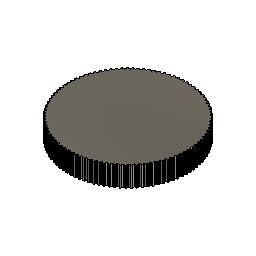
gear_95z (Autodesk Fusion 360 design; units mm, degrees)
Autodesk Fusion 360 part; units mm, degrees
sketch "Sketch1" plane through (0, 0, 0) normal (0, 0, 1) x (1, 0, 0) in component "gt2 pulley"
  circle A0 centre (0, 0) radius 30.2394 construction
  circle A1 centre (0, 0) radius 29.2354 construction
  line L0 (0, 0) -> (0, 30.2394) construction
  line L1 (0, 0) -> (0.9998, 30.2229) construction
  line L2 (0, 0) -> (1.4042, 30.2068) construction
  circle A2 centre (0, 0) radius 29.9854 construction
  arc A3 (0.3977, 29.8499) -> (0.4768, 29.551) centre (1.3924, 29.9531) ccw
  circle A4 centre (0, 0) radius 29.8354 construction
  arc A5 (0.2497, 29.9844) -> (0, 29.9854) centre (0, 0) ccw
  arc A6 (0.3977, 29.8499) -> (0.2497, 29.9844) centre (0.2486, 29.8344) ccw
  arc A7 (0.4768, 29.551) -> (0.9666, 29.2195) centre (0.985, 29.7742) ccw
  arc A8 (0, 29.9854) -> (-0.2497, 29.9844) centre (0, 0) ccw
  arc A9 (-0.2497, 29.9844) -> (-0.3977, 29.8499) centre (-0.2486, 29.8344) ccw
  arc A10 (-0.4768, 29.551) -> (-0.3977, 29.8499) centre (-1.3924, 29.9531) ccw
  arc A11 (-0.9669, 29.2194) -> (-0.4768, 29.551) centre (-0.985, 29.7742) ccw
  arc A12 (0.9666, 29.2195) -> (-0.9666, 29.2195) centre (0, 0) ccw
  point P0 (1.3924, 29.9531)
  point P1 (0, 29.9854)
  dimension "d18" = 60.4789
  dimension "d19" = 1.895
  dimension "d22" = 1.004
  dimension "d24" = 0.75
  dimension "d26" = 1
  dimension "d27" = 0.15
  dimension "d28" = 0.15
  dimension "d47" = 0.555
  dimension "d52" = 3.812
  constraint coincident A0.centre A1.centre
  constraint coincident A0 L0.end
  constraint vertical L0
  constraint coincident A0 L1.end
  constraint coincident A0 L2.end
  constraint concentric A1 A2
  constraint coincident A1 A7.end
  constraint coincident L1 A7.end
  constraint coincident A2 P0
  constraint coincident L2 P0
  constraint coincident P0 A3.centre
  constraint coincident A2 P1
  constraint coincident L0 P1
  constraint concentric A2 A4
  constraint coincident P1 A5.end
  constraint coincident A4 A6.centre
  constraint coincident A3.start A6.start
  constraint tangent A3 A6
  constraint tangent A3 A7
  constraint symmetric L0 A7.end A12.end
  constraint symmetric L0 A3.start A9.end
  constraint symmetric L0 A3.end A10.start
  constraint symmetric L0 A3 A10
  constraint symmetric L0 A5.start A8.end
  constraint symmetric L0 P1 A5.end
  constraint symmetric L0 A5 A8
  constraint symmetric L0 A6 A9
  constraint symmetric L0 A7 A11
  constraint coincident A1 A11.start
  constraint tangent A1 A7
  constraint coincident L1 A7.centre
  measures "d18" diameter of A0
  measures "d19" angle of L0 L1
  measures "d22" distance of A0 A1
  measures "d24" distance of A1 A2
  measures "d26" radius of A3
  measures "d27" distance of A2 A4
  measures "d28" radius of A6
  measures "d47" radius of A7
extrude "Extrude1" add sketch "Sketch1" along normal blind 10 makes body 1
pattern_circular "C-Pattern1" count 95 over 360 about axis through (0, 0, 1.75) along (0, 0, 1) of bodies 1 makes body 2 at (-2.0395, 29.1642, 6.6667) makes body 3 at (-3.1094, 29.0696, 6.6667) makes body 4 at (-6.4983, 28.5041, 6.6667) makes body 5 at (-7.5409, 28.2462, 6.6667) makes body 6 at (-8.7785, 27.8864, 3.3333) makes body 7 at (-11.9894, 26.6639, 6.6667) makes body 8 at (-12.3798, 26.4849, 3.3333) makes body 9 at (-14.6643, 25.2917, 6.6667) makes body 10 at (-16.4817, 24.1467, 6.6667) makes body 11 at (-18.5444, 22.6013, 6.6667) makes body 12 at (-19.9976, 21.3262, 6.6667) makes body 13 at (-20.3087, 21.0302, 3.3333) makes body 14 at (-22.2222, 18.997, 6.6667) makes body 15 at (-22.905, 18.1679, 6.6667) makes body 16 at (-24.0556, 16.6144, 3.3333) makes body 17 at (-25.8387, 13.6775, 6.6667) makes body 18 at (-26.4164, 12.5254, 6.6667) makes body 19 at (-27.4169, 10.1501, 6.6667) makes body 20 at (-27.9659, 8.5217, 6.6667) makes body 21 at (-28.1469, 7.9033, 3.3333) makes body 22 at (-28.6077, 6.0258, 3.3333) makes body 23 at (-29.1171, 2.628, 6.6667) makes body 24 at (-29.2271, 0.6979, 6.6667) makes body 25 at (-29.2342, 0.2685, 6.6667) makes body 26 at (-29.1265, -2.5214, 6.6667) makes body 27 at (-29.0142, -3.5896, 3.3333) makes body 28 at (-28.7136, -5.4993, 3.3333) makes body 29 at (-27.8701, -8.8299, 6.6667) makes body 30 at (-27.7374, -9.2384, 3.3333) makes body 31 at (-26.7296, -11.8422, 6.6667) makes body 32 at (-26.2766, -12.816, 3.3333) makes body 33 at (-25.3722, -14.5246, 3.3333) makes body 34 at (-23.8709, -16.8787, 6.6667) makes body 35 at (-22.2916, -18.9155, 6.6667) makes body 36 at (-22.0113, -19.2409, 3.3333) makes body 37 at (-20.6915, -20.6536, 3.3333) makes body 38 at (-18.627, -22.5332, 6.6667) makes body 39 at (-16.57, -24.0862, 6.6667) makes body 40 at (-15.4923, -24.7931, 6.6667) makes body 41 at (-14.5712, -25.3455, 3.3333) makes body 42 at (-12.0869, -26.6199, 6.6667) makes body 43 at (-9.8979, -27.509, 3.3333) makes body 44 at (-8.4704, -27.9815, 6.6667) makes body 45 at (-7.4369, -28.2737, 3.3333) makes body 46 at (-4.7058, -28.8542, 6.6667) makes body 47 at (-2.7886, -29.1021, 6.6667) makes body 48 at (-0.8591, -29.2228, 6.6667) makes body 49 at (0.2149, -29.2346, 3.3333) makes body 50 at (2.1465, -29.1565, 3.3333) makes body 51 at (4.0688, -28.9509, 3.3333) makes body 52 at (5.9733, -28.6187, 3.3333) makes body 53 at (9.2895, -27.7203, 6.6667) makes body 54 at (11.1013, -27.0458, 6.6667) makes body 55 at (12.8645, -26.2529, 6.6667) makes body 56 at (14.0091, -25.6604, 6.6667) makes body 57 at (14.9421, -25.1285, 3.3333) makes body 58 at (16.5702, -24.0861, 3.3333) makes body 59 at (19.2815, -21.9758, 6.6667) makes body 60 at (20.6917, -20.6534, 6.6667) makes body 61 at (22.0115, -19.2407, 6.6667) makes body 62 at (23.235, -17.7439, 6.6667) makes body 63 at (23.4931, -17.4007, 3.3333) makes body 64 at (24.5918, -15.81, 3.3333) makes body 65 at (26.2768, -12.8157, 6.6667) makes body 66 at (27.0663, -11.0511, 6.6667) makes body 67 at (27.2257, -10.6523, 3.3333) makes body 68 at (27.8702, -8.8296, 3.3333) makes body 69 at (28.3928, -6.9684, 3.3333) makes body 70 at (28.7913, -5.0766, 3.3333) makes body 71 at (29.0639, -3.1627, 3.3333) makes body 72 at (29.233, -0.3758, 6.6667) makes body 73 at (29.2271, 0.6982, 3.3333) makes body 74 at (29.0272, 3.4831, 6.6667) makes body 75 at (28.6076, 6.0261, 6.6667) makes body 76 at (28.516, 6.4457, 3.3333) makes body 77 at (28.0277, 8.3162, 3.3333) makes body 78 at (27.4168, 10.1504, 3.3333) makes body 79 at (26.686, 11.9402, 3.3333) makes body 80 at (25.1009, 14.9885, 6.6667) makes body 81 at (24.4159, 16.0802, 6.6667) makes body 82 at (23.8088, 16.9662, 6.6667) makes body 83 at (22.6354, 18.5026, 3.3333) makes body 84 at (20.3085, 21.0304, 6.6667) makes body 85 at (19.3618, 21.9051, 6.6667) makes body 86 at (18.5441, 22.6014, 3.3333) makes body 87 at (17.0099, 23.7776, 3.3333) makes body 88 at (14.1029, 25.609, 6.6667) makes body 89 at (12.9605, 26.2057, 6.6667) makes body 90 at (10.6021, 27.2453, 6.6667) makes body 91 at (8.7782, 27.8864, 6.6667) makes body 92 at (6.916, 28.4056, 6.6667) makes body 93 at (5.6573, 28.6829, 6.6667) makes body 94 at (4.5999, 28.8713, 3.3333) makes body 95 at (1.8248, 29.1784, 6.6667)
sketch "Sketch2" plane through (0, 0, 10) normal (0, 0, 1) x (-1, 0, 0)
  arc A0 (-13.6871, -26.5299) -> (-13.6147, -26.7164) centre (-13.5467, -26.5827) ccw
  arc A1 (-13.6147, -26.7164) -> (-13.1679, -26.9395) centre (0, 0) ccw
  arc A2 (-13.1679, -26.9395) -> (-12.9753, -26.8852) centre (-13.1019, -26.8047) ccw
  arc A3 (-12.7711, -26.6531) -> (-12.9753, -26.8852) centre (-12.1315, -27.4218) ccw
  arc A4 (-12.1848, -26.5752) -> (-12.7711, -26.6531) centre (-12.4161, -27.0797) ccw
  arc A5 (-13.9145, -25.7118) -> (-12.1848, -26.5752) centre (0, 0) ccw
  arc A6 (-13.6244, -26.2272) -> (-13.9145, -25.7118) centre (-14.1787, -26.1999) ccw
  arc A7 (-13.6871, -26.5299) -> (-13.6244, -26.2272) centre (-14.6231, -26.178) ccw
  circle A8 centre (0, 0) radius 29.2354
  constraint coincident A1.centre A5.centre
extrude "Extrude2" add sketch "Sketch2" against normal blind 10 contours A5 A8 bodies 1 2 3 4 5 6 7 8 9 10 11 12 13 14 15 16 17 18 19 20 21 22 23 24 25 26 27 28 29 30 31 32 33 34 35 36 37 38 39 40 41 42 43 44 45 46 47 48 49 50 51 52 53 54 55 56 57 58 59 60 61 62 63 64 65 66 67 68 69 70 71 72 73 74 75 76 77 78 79 80 81 82 83 84 85 86 87 88 89 90 91 92 93 94 95
extrude "Extrude4" [suppressed] in component "gt2 pulley"
pattern_circular "C-Pattern7" [suppressed] in component "gt2 pulley"
extrude "Extrude3" [suppressed] in component "gt2 pulley"
pattern_circular "C-Pattern6" [suppressed] in component "gt2 pulley"
extrude "Extrude2'" [suppressed] in component "gt2 pulley"
pattern_circular "C-Pattern5" [suppressed] in component "gt2 pulley"
extrude "Extrude1'" [suppressed] in component "gt2 pulley"
pattern_circular "C-Pattern4" [suppressed] in component "gt2 pulley"
pattern_circular "C-Pattern3" [suppressed] in component "gt2 pulley"
pattern_circular "C-Pattern2" [suppressed] in component "gt2 pulley"
pattern_circular "C-Pattern1'" [suppressed] in component "gt2 pulley"
copy_body "Body->Comp1" [suppressed] in component "Component"
copy_body "Body->Comp2" [suppressed] in component "Component'"
copy_body "Body->Comp3" [suppressed] in component "Component''"
copy_body "Body->Comp4" [suppressed] in component "Component'''"
copy_body "Body->Comp5" [suppressed] in component "Component''''"
copy_body "Body->Comp6" [suppressed] in component "Component'''''"
copy_body "Body->Comp7" [suppressed] in component "Component''''''"
copy_body "Body->Comp8" [suppressed] in component "Component'''''''"
copy_body "Body->Comp9" [suppressed] in component "Component''''''''"
copy_body "Body->Comp10" [suppressed] in component "Component'''''''''"
copy_body "Body->Comp11" [suppressed] in component "Component''''''''''"
copy_body "Body->Comp12" [suppressed] in component "Component'''''''''''"
copy_body "Body->Comp13" [suppressed] in component "Component''''''''''''"
copy_body "Body->Comp14" [suppressed] in component "Component'''''''''''''"
copy_body "Body->Comp15" [suppressed] in component "Component''''''''''''''"
copy_body "Body->Comp16" [suppressed] in component "Component'''''''''''''''"
copy_body "Body->Comp17" [suppressed] in component "Component''''''''''''''''"
copy_body "Body->Comp18" [suppressed] in component "Component'''''''''''''''''"
copy_body "Body->Comp19" [suppressed] in component "Component''''''''''''''''''"
copy_body "Body->Comp20" [suppressed] in component "Component'''''''''''''''''''"
component "gt2 pulley" placed x (1, 0, 0) y (0, 1, 0) z (0, 0, 1) at (0, 0, 0)
equation "NumTeeth = 95" comment "min 20"
equation "ToothPitch = 2 mm"
equation "PullyDia = NumTeeth * ToothPitch / PI"
equation "ToothAng = ( ( 360 / NumTeeth ) * 1 deg )"
equation "TransOffsetAngle = ToothAng * 0.2"
equation "Sholulder_Radius = 0.15 mm"
equation "Root_Radius = 0.555 mm"
equation "TransRadius = 1 mm"
equation "ToolHeight = 0.75 mm"
equation "PLD = 0.254 mm"
equation "d18 = PullyDia"
equation "d19 = ToothAng / 2"
equation "d22 = PLD + ToolHeight"
equation "d24 = ToolHeight"
equation "d26 = TransRadius"
equation "d27 = Sholulder_Radius"
equation "d31 = NumTeeth"
equation "d33 = NumTeeth"
equation "d35 = NumTeeth"
equation "d37 = NumTeeth"
equation "d41 = NumTeeth"
equation "d45 = NumTeeth"
equation "d47 = Root_Radius"
equation "d50 = NumTeeth"
